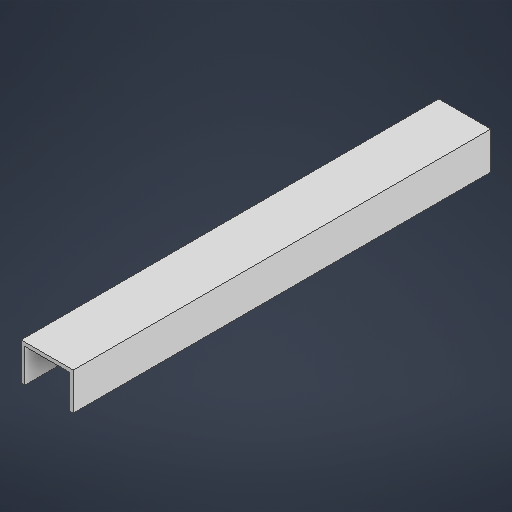
# Autodesk Inventor part: fan_duct
Saved by Autodesk Inventor 2027.1 (Build 311270010, 270A)
## iProperties
Created: 2026-10-02
Part Number: fan_duct
Material: Generic
Document SubType Name: Modeling
Designer: Arik
Density: 1 g/cm^3
Appearance: Default
Author: Arik
Autodesk Inventor part; units mm, degrees
ref_plane "YZ Plane" through (0, 0, 0) normal (1, 0, 0) x (0, 1, 0)
ref_plane "XZ Plane" through (0, 0, 0) normal (0, 1, 0) x (-1, 0, 0)
ref_plane "XY Plane" through (0, 0, 0) normal (0, 0, 1) x (1, 0, 0)
sketch "Sketch1" plane through (0, 0, 0) normal (0, 0, 1) x (1, 0, 0)
  line L0 (0, 0) -> (28, 0)
  line L1 (28, 0) -> (28, 20)
  line L2 (28, 20) -> (0, 20)
  line L3 (0, 20) -> (0, 0)
  line L4 (2, 18) -> (26, 18)
  line L5 (26, 18) -> (26, 2)
  line L6 (26, 2) -> (2, 2)
  line L7 (2, 2) -> (2, 18)
  line L8 (2, 2) -> (2, 0)
  line L9 (26, 2) -> (26, 0)
  dimension "d0" = 28
  dimension "d1" = 20
  dimension "d2" = 2
  constraints: 20 end point, 4 parallel, 4 perpendicular, 2 point on line, 1 horizontal, 3 other
  measures "d0" distance of L2.end L1.end
  measures "d1" distance of L1.end L0.end
  measures "d2" distance between parallel lines of L2 L4
extrude "Extrusion1" add sketch "Sketch1" along normal blind 220 contours L3 L2 L1 L0 L9 L5 L4 L7 L8
sketch "Sketch2" plane through (0, 0, 0) normal (0, 0, -1) x (-1, 0, 0)
  line L0 (-28, 20) -> (0, 20) projected
  line L1 (0, 0) -> (-2, 0) projected
  line L2 (-28, 20) -> (0, 20)
  line L3 (0, 20) -> (0, 0)
  line L4 (0, 0) -> (-28, 0)
  line L5 (-28, 0) -> (-28, 20)
  constraints: 8 end point, 2 parallel, 1 horizontal, 1 perpendicular
extrude "Extrusion2" add sketch "Sketch2" along normal blind 4
body "Solid1"
